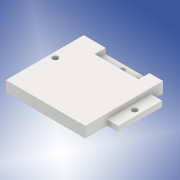
# Autodesk Inventor part: SP002
Saved by Autodesk Inventor 2017 SP1 (Build 210196100, 196)
## iProperties
Created: 2017-08-09
Part Number: SP002
Material: ABS Plastic
Document SubType Name: Modeling
Designer: Zach
Density: 1.06 g/cm^3
Appearance: CR White
Author: Zach
Autodesk Inventor part; units mm, degrees
ref_plane "YZ Plane" through (0, 0, 0) normal (1, 0, 0) x (0, 1, 0)
ref_plane "XZ Plane" through (0, 0, 0) normal (0, 1, 0) x (-1, 0, 0)
ref_plane "XY Plane" through (0, 0, 0) normal (0, 0, 1) x (1, 0, 0)
sketch "Sketch1" plane through (0, 0, 0) normal (0, 0, 1) x (1, 0, 0)
  line L0 (0, 0) -> (72.4, 0)
  line L1 (72.4, 0) -> (72.4, 71)
  line L2 (72.4, 71) -> (0, 71)
  line L3 (0, 71) -> (0, 0)
  dimension "d0" = 72.4
  dimension "d1" = 71
  constraints: 8 end point, 2 parallel, 1 horizontal, 1 perpendicular
  measures "d0" distance of L2.end L1.end
  measures "d1" distance of L0.end L1.end
extrude "Extrusion1" add sketch "Sketch1" along normal blind 10
sketch "Sketch2" plane through (0, 0, 10) normal (0, 0, 1) x (1, 0, 0)
  line L0 (72.4, 0) -> (72.4, 71) projected
  line L1 (72.4, 20) -> (82.4, 20)
  line L2 (82.4, 20) -> (82.4, 60)
  line L3 (82.4, 60) -> (72.4, 60)
  line L4 (72.4, 60) -> (72.4, 20)
  line L5 (72.4, 71) -> (0, 71) projected
  circle A0 centre (77.4, 40) radius 2.5
  line L6 (0, 0) -> (72.4, 0) projected
  point P0 (82.4, 40)
  point P1 (77.4, 60)
  dimension "d4" = 10
  dimension "d5" = 40
  dimension "d7" = 5
  dimension "d22" = 20
  constraints: 8 end point, 2 midpoint, 2 parallel, 1 centre point, 1 horizontal, 1 horizontal alignment, 1 perpendicular, 1 point on line, 1 vertical alignment
  measures "d4" distance of L3.end L2.end
  measures "d5" distance of L2.end L1.end
  measures "d7" diameter of A0
  measures "d22" distance between parallel lines of L6 L1
extrude "Extrusion2" add sketch "Sketch2" against normal blind 10
sketch "Sketch3" plane through (0, 0, 10) normal (0, 0, 1) x (1, 0, 0)
  line L0 (72.4, 60) -> (82.4, 60) projected
  line L1 (72.4, 20) -> (82.4, 20) projected
  line L2 (82.4, 60) -> (72.4, 60)
  line L3 (72.4, 60) -> (72.4, 20)
  line L4 (72.4, 20) -> (82.4, 20)
  line L5 (82.4, 20) -> (82.4, 60)
  point P0 (0, 0)
  constraints: 8 end point, 2 parallel, 1 horizontal, 1 perpendicular
extrude "Extrusion3" cut sketch "Sketch3" against normal blind 5
sketch "Sketch4" plane through (0, 0, 0) normal (0, 0, -1) x (-1, 0, 0)
  line L0 (0, 71) -> (0, 0) projected
  line L1 (0, 60) -> (-10, 60)
  line L2 (-10, 60) -> (-10, 20)
  line L3 (-10, 20) -> (0, 20)
  line L4 (0, 20) -> (0, 60)
  point P0 (-72.4, 60)
  dimension "d15" = 10
  dimension "d16" = 40
  constraints: 8 end point, 2 parallel, 1 horizontal, 1 horizontal alignment, 1 perpendicular, 1 point on line
  measures "d15" distance of L3.end L2.end
  measures "d16" distance of L2.end L1.end
extrude "Extrusion4" cut sketch "Sketch4" against normal blind 5
sketch "Sketch5" plane through (0, 0, 5) normal (0, 0, -1) x (-1, 0, 0)
  circle A0 centre (-5, 40) radius 2.5
  line L0 (0, 60) -> (0, 20) projected
  line L1 (-10, 60) -> (0, 60) projected
  point P0 (0, 0)
  point P1 (0, 40)
  point P2 (-5, 60)
  dimension "d19" = 5
  constraints: 2 midpoint, 1 centre point, 1 horizontal alignment, 1 vertical alignment
  measures "d19" diameter of A0
extrude "Extrusion5" cut sketch "Sketch5" against normal through all
sketch "Sketch6" plane through (0, 0, 10) normal (0, 0, 1) x (1, 0, 0)
  line L0 (72.4, 71) -> (0, 71) projected
  line L1 (60, 71) -> (20, 71)
  line L2 (20, 71) -> (20, 61)
  line L3 (20, 61) -> (60, 61)
  line L4 (60, 61) -> (60, 71)
  line L5 (0, 71) -> (0, 0) projected
  dimension "d23" = 40
  dimension "d24" = 10
  dimension "d25" = 20
  constraints: 8 end point, 2 parallel, 1 horizontal, 1 perpendicular, 1 point on line
  measures "d23" distance of L3.end L2.end
  measures "d24" distance of L2.end L1.end
  measures "d25" distance between parallel lines of L5 L2
extrude "Extrusion6" cut sketch "Sketch6" against normal blind 5
sketch "Sketch7" plane through (0, 0, 5) normal (0, 0, 1) x (1, 0, 0)
  circle A0 centre (40, 66) radius 2.5
  line L0 (60, 61) -> (20, 61) projected
  line L1 (20, 61) -> (20, 71) projected
  point P0 (0, 0)
  point P1 (40, 61)
  point P2 (20, 66)
  dimension "d28" = 5
  constraints: 2 midpoint, 1 centre point, 1 horizontal alignment, 1 vertical alignment
  measures "d28" diameter of A0
extrude "Extrusion7" cut sketch "Sketch7" against normal through all
body "Solid1"
